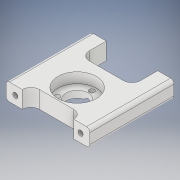
# Autodesk Inventor part: Motorhalterung leicht versuch dünn
Saved by Autodesk Inventor 2018 (Build 220112000, 112)
## iProperties
Created: 2019-03-03
Part Number: Motorhalterung leicht versuch dünn
Material: ABS-Kunststoff
Document SubType Name: Modeling
Designer: RedBots
Density: 0.455903 g/cm^3
Appearance: Weiß
Mass: 11 g
Surface Area: 91.5152 cm^2
Volume: 24.1279 cm^3
Author: RedBots
Autodesk Inventor part; units mm, degrees
ref_plane "YZ Plane" through (0, 0, 0) normal (1, 0, 0) x (0, 1, 0)
ref_plane "XZ Plane" through (0, 0, 0) normal (0, 1, 0) x (-1, 0, 0)
ref_plane "XY Plane" through (0, 0, 0) normal (0, 0, 1) x (1, 0, 0)
sketch "Skizze2" plane through (0, 0, 0) normal (0, 0, 1) x (1, 0, 0)
  line L0 (0, 0) -> (49, 0)
  line L1 (0, 0) -> (49, 0) construction
  line L2 (49, 0) -> (49, 49)
  line L3 (49, 49) -> (0, 49)
  line L4 (0, 49) -> (0, 0)
  dimension "d16" = 49
  dimension "d18" = 49
  constraints: 10 end point, 2 equal length, 2 horizontal, 2 perpendicular
  measures "d16" distance of L0.start L0.end
  measures "d18" distance of L0.end L2.end
extrude "Extrusion1" add sketch "Skizze2" along normal blind 10
sketch "Skizze3" plane through (0, 0, 10) normal (0, 0, 1) x (1, 0, 0)
  circle A0 centre (24.5, 17) radius 11.25
  line L0 (0, 49) -> (0, 0) construction
  line L1 (0, 17) -> (49, 17) construction
  line L2 (49, 0) -> (49, 49) construction
  line L3 (0, 0) -> (49, 0) construction
  dimension "d72" = 22.5
  dimension "d73" = 17
  constraints: 2 end point, 2 point on line, 1 centre point, 1 coincident, 1 horizontal, 1 midpoint
  measures "d72" diameter of A0
  measures "d73" distance between parallel lines of L3 L1
extrude "Extrusion2" cut sketch "Skizze3" against normal blind 6
sketch "Skizze4" plane through (24.5, 17, 4) normal (0, 0, 1) x (1, 0, 0)
  circle A0 centre (7.3612, -4.25) radius 1.5
  circle A1 centre (0, 8.5) radius 1.5
  circle A2 centre (-7.3612, -4.25) radius 1.5
  line L0 (0, 0) -> (0, 8.5) construction
  line L1 (-24.5, -17) -> (24.5, -17) construction
  circle A3 centre (0, 0) radius 11.25 construction
  line L2 (0, -17) -> (0, 0) construction
  line L3 (0, 0) -> (7.3612, -4.25) construction
  line L4 (0, 0) -> (-7.3612, -4.25) construction
  circle A4 centre (0, 0) radius 6.5
  dimension "d37" = 3
  dimension "d42" = 3
  dimension "d43" = 3
  dimension "d90" = 8.5
  dimension "d91" = 120
  dimension "d92" = 120
  dimension "d93" = 13
  constraints: 8 end point, 4 centre point, 4 coincident, 2 equal length, 2 vertical, 1 midpoint
  measures "d37" diameter of A0
  measures "d42" diameter of A1
  measures "d43" diameter of A2
  measures "d90" distance of L0.start L0.end
  measures "d91" angle of L3 L0
  measures "d92" angle of L0 L4
  measures "d93" diameter of A4
extrude "Extrusion3" cut sketch "Skizze4" against normal up to next
sketch "Skizze9" plane through (0, 49, 0) normal (0, 1, 0) x (1, 0, 0)
  line L0 (24.5, -5) -> (43.5, -5) construction
  circle A0 centre (5.5, -5) radius 1.5
  circle A1 centre (43.5, -5) radius 1.5
  line L1 (0, -10) -> (49, -10) construction
  line L2 (24.5, -10) -> (24.5, 0) construction
  line L3 (49, 0) -> (0, 0) construction
  line L4 (5.5, -5) -> (24.5, -5) construction
  dimension "d58" = 3
  dimension "d89" = 19
  constraints: 7 end point, 3 midpoint, 2 centre point, 2 collinear, 1 coincident, 1 equal radius, 1 horizontal, 1 vertical
  measures "d58" diameter of A0
  measures "d89" distance of L0.start L0.end
extrude "Extrusion6" cut sketch "Skizze9" against normal blind 56
sketch "Skizze12" plane through (0, 0, 0) normal (0, 0, -1) x (-1, 0, 0)
  circle A0 centre (-24.5, 25.5) radius 1.5 projected
  circle A1 centre (-24.5, 25.5) radius 3
  circle A2 centre (-17.1388, 12.75) radius 1.5 projected
  circle A3 centre (-17.1388, 12.75) radius 3
  circle A4 centre (-31.8612, 12.75) radius 1.5 projected
  circle A5 centre (-31.8612, 12.75) radius 3
  point P0 (0, 0)
  dimension "d80" = 6
  dimension "d81" = 6
  dimension "d82" = 6
  constraints: 3 centre point, 3 coincident
  measures "d80" diameter of A1
  measures "d81" diameter of A3
  measures "d82" diameter of A5
extrude "Extrusion8" cut sketch "Skizze12" against normal blind 0.16
chamfer "Fase3" distance 1.5 angle 45 3 edges at (23, 25.5, 0.16) (30.3612, 12.75, 0.16) (15.6388, 12.75, 0.16)
fillet "Rundung2" radius 0.5 3 edges at (23, 25.5, 1.66) (30.3612, 12.75, 1.66) (15.6388, 12.75, 1.66)
sketch "Skizze14" plane through (0, 0, 0) normal (0, 0, -1) x (-1, 0, 0)
  line L0 (-39.5, 49) -> (-9.5, 49)
  line L1 (-9.5, 49) -> (-9.5, 34)
  line L2 (-9.5, 34) -> (-39.5, 34)
  line L3 (-39.5, 34) -> (-39.5, 49)
  line L4 (-49, 49) -> (0, 49) projected
  line L5 (-49, 0) -> (-49, 49) construction
  line L6 (0, 49) -> (0, 0) construction
  line L7 (-39.5, 0) -> (-9.5, 0)
  line L8 (-9.5, 0) -> (-9.5, 5)
  line L9 (-9.5, 5) -> (-39.5, 5)
  line L10 (-39.5, 5) -> (-39.5, 0)
  line L11 (0, 0) -> (-49, 0) projected
  point P0 (-24.5, 49)
  point P1 (-24.5, 0)
  point P2 (-24.5, 0)
  dimension "d95" = 15
  dimension "d96" = 30
  dimension "d101" = 5
  constraints: 16 end point, 6 midpoint, 3 horizontal, 3 parallel, 2 vertical, 1 perpendicular
  measures "d95" distance of L0.end L1.end
  measures "d96" distance between parallel lines of L1 L3
  measures "d101" distance of L7.end L9.start
extrude "Extrusion9" cut sketch "Skizze14" against normal up to next
fillet "Rundung3" radius 5 4 edges at (39.5, 34, 5) (9.5, 34, 5) (39.5, 5, 5) (9.5, 5, 5)
fillet "Rundung4" radius 2 4 edges at (49, 24.5, 10) (49, 24.5, 0) (0, 24.5, 0) (0, 24.5, 10)
